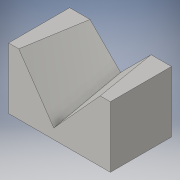
# Autodesk Inventor part: loft cut cordier
Saved by Autodesk Inventor 2016 (Build 200138000, 138)
## iProperties
Created: 2017-01-18
Part Number: loft cut cordier
Material: Generic
Document SubType Name: Modeling
Designer: 170007
Density: 1 g/cm^3
Appearance: Default
Author: 170007
Autodesk Inventor part; units mm, degrees
ref_plane "YZ Plane" through (0, 0, 0) normal (1, 0, 0) x (0, 1, 0)
ref_plane "XZ Plane" through (0, 0, 0) normal (0, 1, 0) x (-1, 0, 0)
ref_plane "XY Plane" through (0, 0, 0) normal (0, 0, 1) x (1, 0, 0)
sketch "Sketch1" plane through (0, 0, 0) normal (0, 0, 1) x (1, 0, 0)
  line L0 (0, 0) -> (63.5, 0)
  line L1 (63.5, 0) -> (63.5, 38.1)
  line L2 (63.5, 38.1) -> (0, 38.1)
  line L3 (0, 38.1) -> (0, 0)
  dimension "d0" = 63.5
  dimension "d1" = 38.1
  constraints: 8 end point, 2 parallel, 1 horizontal, 1 perpendicular
  measures "d0" distance of L2.end L1.end
  measures "d1" distance of L1.end L0.end
extrude "Extrusion1" add sketch "Sketch1" along normal blind 38.1
sketch "Sketch2" plane through (0, 0, 38.1) normal (0, 0, 1) x (1, 0, 0)
  line L0 (63.5, 38.1) -> (0, 38.1) projected
  line L1 (6.35, 38.1) -> (28.2442, 6.35)
  line L2 (28.2442, 6.35) -> (57.15, 38.1)
  line L3 (0, 0) -> (63.5, 0) projected
  line L4 (6.35, 38.1) -> (57.15, 38.1)
  dimension "d4" = 6.35
  dimension "d5" = 6.35
  dimension "d6" = 6.35
  constraints: 6 end point, 2 point on line, 1 horizontal
  measures "d4" distance of L0.end L1.start
  measures "d5" distance from line of L3 L1.end
  measures "d6" distance of L0.start L2.end
sketch "Sketch3" plane through (0, 0, 0) normal (0, 0, -1) x (-1, 0, 0)
  line L0 (-63.5, 38.1) -> (0, 38.1) projected
  line L1 (-50.8, 38.1) -> (-31.75, 19.05)
  line L2 (-31.75, 19.05) -> (-12.7, 38.1)
  line L3 (0, 0) -> (-63.5, 0) projected
  line L4 (0, 38.1) -> (0, 0) projected
  line L5 (-50.8, 38.1) -> (-12.7, 38.1)
  dimension "d7" = 12.7
  dimension "d8" = 19.05
  dimension "d9" = 12.7
  dimension "d10" = 31.75
  constraints: 6 end point, 2 point on line, 1 collinear
  measures "d7" distance of L0.start L1.start
  measures "d8" distance from line of L3 L1.end
  measures "d9" distance of L0.end L2.end
  measures "d10" distance from line of L4 L1.end
loft "Loft1" cut profiles "Sketch2", "Sketch3"
body "Solid1"
